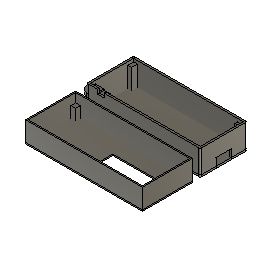
Asksin XS Board (Autodesk Fusion 360 design; units mm, degrees)
Autodesk Fusion 360 part; units mm, degrees
sketch "Skizze1" plane through (0, 0, 0) normal (0, 0, 1) x (1, 0, 0)
  line L0 (0.0871, 28.0002) -> (59.7871, 28.0002)
  line L1 (59.7871, 28.0002) -> (59.7871, 3.4002)
  line L2 (59.7871, 3.4002) -> (0.0871, 3.4002)
  line L3 (0.0871, 3.4002) -> (0.0871, 28.0002)
  line L4 (58.7871, 4.4002) -> (1.0871, 4.4002)
  line L5 (1.0871, 4.4002) -> (1.0871, 27.0002)
  line L6 (1.0871, 27.0002) -> (58.7871, 27.0002)
  line L7 (58.7871, 27.0002) -> (58.7871, 4.4002)
  line L8 (1.0871, 27.0002) -> (3.0871, 27.0002)
  line L9 (3.0871, 27.0002) -> (3.0871, 24.0002)
  line L10 (3.0871, 24.0002) -> (1.0871, 24.0002)
  line L11 (1.0871, 24.0002) -> (1.0871, 27.0002)
  line L12 (1.0871, 4.4002) -> (9.0871, 4.4002)
  line L13 (9.0871, 4.4002) -> (9.0871, 6.9002)
  line L14 (9.0871, 6.9002) -> (1.0871, 6.9002)
  line L15 (1.0871, 6.9002) -> (1.0871, 4.4002)
  line L16 (58.7871, 27.0002) -> (55.7871, 27.0002)
  line L17 (55.7871, 27.0002) -> (55.7871, 25.5002)
  line L18 (55.7871, 25.5002) -> (58.7871, 25.5002)
  line L19 (58.7871, 25.5002) -> (58.7871, 27.0002)
  line L20 (58.7871, 4.4002) -> (55.7871, 4.4002)
  line L21 (55.7871, 4.4002) -> (55.7871, 5.9002)
  line L22 (55.7871, 5.9002) -> (58.7871, 5.9002)
  line L23 (58.7871, 5.9002) -> (58.7871, 4.4002)
  line L24 (58.7871, 19.7002) -> (59.7871, 19.7002)
  line L25 (59.7871, 19.7002) -> (59.7871, 11.7002)
  line L26 (59.7871, 11.7002) -> (58.7871, 11.7002)
  line L27 (58.7871, 11.7002) -> (58.7871, 19.7002)
  circle A0 centre (-5.1629, 15.7002) radius 1.75
  line L28 (0.0871, 20.9502) -> (-6.9129, 20.9502)
  line L29 (-10.4129, 17.4502) -> (-10.4129, 13.9502)
  line L30 (-6.9129, 10.4502) -> (0.0871, 10.4502)
  line L31 (0.0871, 10.4502) -> (0.0871, 20.9502)
  arc A1 (-6.9129, 20.9502) -> (-10.4129, 17.4502) centre (-6.9129, 17.4502) ccw
  arc A2 (-10.4129, 13.9502) -> (-6.9129, 10.4502) centre (-6.9129, 13.9502) ccw
  point P0 (-10.4129, 20.9502)
  point P1 (-5.1629, 20.9502)
  point P2 (-10.4129, 15.7002)
  point P3 (0.0871, 15.7002)
  dimension "d1" = 59.7
  dimension "d2" = 24.6
  dimension "d3" = 1
  dimension "d4" = 2
  dimension "d5" = 3
  dimension "d6" = 8
  dimension "d7" = 2.5
  dimension "d8" = 3
  dimension "d9" = 1.5
  dimension "d10" = 3
  dimension "d11" = 1.5
  dimension "d12" = 1
  dimension "d13" = 8
  dimension "d14" = 8.3
  dimension "d57" = 3.5
  dimension "d58" = 10.5
  dimension "d59" = 10.5
  dimension "d60" = 3.5
  constraint horizontal L0
  constraint vertical L1
  constraint horizontal L2
  constraint vertical L3
  constraint horizontal L8
  constraint vertical L9
  constraint horizontal L10
  constraint vertical L11
  constraint horizontal L12
  constraint vertical L13
  constraint horizontal L14
  constraint vertical L15
  constraint horizontal L16
  constraint vertical L17
  constraint horizontal L18
  constraint vertical L19
  constraint horizontal L20
  constraint vertical L21
  constraint horizontal L22
  constraint vertical L23
  constraint horizontal L24
  constraint vertical L25
  constraint horizontal L26
  constraint vertical L27
  constraint coincident L7 L24.start
  constraint horizontal L28
  constraint vertical L29
  constraint horizontal L30
  constraint vertical L31
  constraint coincident L3 L28.start
  constraint vertical A0.centre P1
  constraint horizontal A0.centre P2
  constraint midpoint L3 P3
  constraint horizontal A0.centre P3
  constraint coincident L28 P1
  constraint coincident L29 P2
  constraint coincident P0 L28
  constraint coincident P0 L29
  constraint tangent L28 A1
  constraint tangent L29 A1
  constraint tangent L29 A2
  constraint tangent L30 A2
  constraint equal A1 A2
  measures "d1" distance of L0.start L0.end
  measures "d2" distance of L0.start L2.end
  measures "d4" distance of L5.end L8.end
  measures "d5" distance of L5.end L10.end
  measures "d6" distance of L4.end L12.end
  measures "d7" distance of L4.end L14.end
  measures "d8" distance of L6.end L16.end
  measures "d9" distance of L6.end L18.end
  measures "d10" distance of L4.start L20.end
  measures "d11" distance of L4.start L22.end
  measures "d12" distance of L24.start L24.end
  measures "d13" distance of L24.start L26.end
  measures "d14" distance of L0 L24
  measures "d57" diameter of A0
  measures "d58" distance of L28.start P0
  measures "d59" distance of L28.start L30.end
  measures "d60" radius of A1
extrude "Extrusion1" add sketch "Skizze1" along normal blind 1 contours L0 L1 L2 L3 L4 L5 L6 L7 L8 L11 L12 L15 L16 L19 L20 L23 L24 L26 L31 | L1 L7 L24 L25 L26 L27 | L4 L5 L6 L7 L9 L10 L13 L14 L17 L18 L21 L22 L27 | L6 L7 L16 L17 L18 L19 | L4 L7 L20 L21 L22 L23 | L5 L6 L8 L9 L10 L11 | L4 L5 L12 L13 L14 L15 makes body 1
extrude "Extrusion3" add sketch "Skizze1" along normal blind 13.2 separate body contours L0 L1 L2 L3 L4 L5 L6 L7 L8 L11 L12 L15 L16 L19 L20 L23 L24 L26 L31 | L1 L7 L24 L25 L26 L27 makes body 2
extrude "Extrusion4" cut sketch "Skizze1" along normal blind 5 contours L1 L7 L24 L25 L26 L27 bodies 2
sketch "Skizze2" plane through (0, 0, 0) normal (0, 0, 1) x (1, 0, 0)
  line L0 (59.9433, -27.2284) -> (-1.5067, -27.2284)
  line L1 (-1.5067, -27.2284) -> (-1.5067, -0.9284)
  line L2 (-1.5067, -0.9284) -> (59.9433, -0.9284)
  line L3 (59.9433, -0.9284) -> (59.9433, -27.2284)
  line L4 (-0.8067, -1.6284) -> (59.2433, -1.6284)
  line L5 (59.2433, -1.6284) -> (59.2433, -26.5284)
  line L6 (59.2433, -26.5284) -> (-0.8067, -26.5284)
  line L7 (-0.8067, -26.5284) -> (-0.8067, -1.6284)
  line L8 (26.7433, -9.5784) -> (51.7433, -9.5784)
  line L9 (51.7433, -9.5784) -> (51.7433, -18.5784)
  line L10 (51.7433, -18.5784) -> (26.7433, -18.5784)
  line L11 (26.7433, -18.5784) -> (26.7433, -9.5784)
  line L12 (-0.8067, -1.6284) -> (1.6933, -1.6284)
  line L13 (1.6933, -1.6284) -> (1.6933, -4.1284)
  line L14 (1.6933, -4.1284) -> (-0.8067, -4.1284)
  line L15 (-0.8067, -4.1284) -> (-0.8067, -1.6284)
  line L16 (-0.8067, -26.5284) -> (1.6933, -26.5284)
  line L17 (1.6933, -26.5284) -> (1.6933, -24.0284)
  line L18 (1.6933, -24.0284) -> (-0.8067, -24.0284)
  line L19 (-0.8067, -24.0284) -> (-0.8067, -26.5284)
  line L20 (59.2433, -1.6284) -> (56.7433, -1.6284)
  line L21 (56.7433, -1.6284) -> (56.7433, -4.1284)
  line L22 (56.7433, -4.1284) -> (59.2433, -4.1284)
  line L23 (59.2433, -4.1284) -> (59.2433, -1.6284)
  line L24 (59.2433, -26.5284) -> (56.7433, -26.5284)
  line L25 (56.7433, -26.5284) -> (56.7433, -24.0284)
  line L26 (56.7433, -24.0284) -> (59.2433, -24.0284)
  line L27 (59.2433, -24.0284) -> (59.2433, -26.5284)
  dimension "d23" = 61.45
  dimension "d24" = 26.3
  dimension "d26" = 0.7
  dimension "d27" = 25
  dimension "d28" = 9
  dimension "d29" = 8.65
  dimension "d30" = 7.5
  dimension "d37" = 2.5
  dimension "d38" = 2.5
  dimension "d39" = 2.5
  dimension "d40" = 2.5
  dimension "d41" = 2.5
  dimension "d42" = 2.5
  dimension "d43" = 2.5
  dimension "d44" = 2.5
  dimension "d63" = 24.5
  dimension "d64" = 59.5
  dimension "d65" = 7.4
  constraint horizontal L2
  constraint vertical L3
  constraint horizontal L0
  constraint vertical L1
  constraint horizontal L8
  constraint vertical L9
  constraint horizontal L10
  constraint vertical L11
  constraint horizontal L12
  constraint vertical L13
  constraint horizontal L14
  constraint vertical L15
  constraint horizontal L16
  constraint vertical L17
  constraint horizontal L18
  constraint vertical L19
  constraint horizontal L20
  constraint vertical L21
  constraint horizontal L22
  constraint vertical L23
  constraint horizontal L24
  constraint vertical L25
  constraint horizontal L26
  constraint vertical L27
  measures "d23" distance of L2.end L1.end
  measures "d24" distance of L1.end L0.end
  measures "d27" distance of L8.start L8.end
  measures "d28" distance of L8.start L10.end
  measures "d29" distance of L2 L8
  measures "d30" distance of L5 L9
  measures "d37" distance of L4.start L12.end
  measures "d38" distance of L4.start L14.end
  measures "d39" distance of L6.end L16.end
  measures "d40" distance of L6.end L18.end
  measures "d41" distance of L4.end L20.end
  measures "d42" distance of L4.end L22.end
  measures "d43" distance of L5.end L24.end
  measures "d44" distance of L5.end L26.end
extrude "Extrusion5" add sketch "Skizze2" along normal blind 0.7 separate body contours L0 L1 L2 L3 | L4 L7 L12 L13 L14 L15 | L4 L5 L6 L7 L13 L14 L17 L18 L21 L22 L25 L26 | L4 L5 L20 L21 L22 L23 | L6 L7 L16 L17 L18 L19 | L5 L6 L24 L25 L26 L27 makes body 3
extrude "Extrusion6" add sketch "Skizze2" along normal blind 11 separate body contours L0 L1 L2 L3 makes body 4
extrude "Extrusion7" add sketch "Skizze1" along normal blind 11.6 separate body contours L6 L7 L16 L17 L18 L19 | L4 L7 L20 L21 L22 L23 | L5 L6 L8 L9 L10 L11 | L4 L5 L12 L13 L14 L15 makes body 5 at (56.7871, 27.0002, 3.8667) makes body 6 at (57.7871, 4.4002, 3.8667) makes body 7 at (1.0871, 25.0002, 3.8667) makes body 8 at (6.4204, 6.9002, 3.8667)
extrude "Extrusion8" add sketch "Skizze2" along normal blind 6.3 separate body contours L4 L7 L12 L13 L14 L15 | L4 L5 L20 L21 L22 L23 | L6 L7 L16 L17 L18 L19 | L5 L6 L24 L25 L26 L27 makes body 9 at (0.0266, -1.6284, 2.1) makes body 10 at (0.86, -24.0284, 2.1) makes body 11 at (59.2433, -2.4617, 2.1) makes body 12 at (58.41, -26.5284, 2.1)
fillet "Abrundung1" radius 0.7 1 edges at (0.0871, 28.0002, 6.6) on bodies 2
fillet "Abrundung2" radius 0.7 1 edges at (0.0871, 28.0002, 0.5) on bodies 1
fillet "Abrundung3" radius 0.7 2 edges at (0.0871, 3.4002, 0.5) (0.0871, 3.4002, 6.6) on bodies 1 2
fillet "Abrundung4" radius 0.7 1 edges at (59.7871, 28.0002, 6.6) on bodies 2
fillet "Abrundung5" radius 0.7 1 edges at (59.7871, 28.0002, 0.5) on bodies 1
fillet "Abrundung6" radius 0.7 2 edges at (59.7871, 3.4002, 0.5) (59.7871, 3.4002, 6.6) on bodies 1 2
sketch "Skizze3" plane through (0, 3.4002, 0) normal (0, -1, 0) x (1, 0, 0)
  line L0 (59.0871, 0) -> (59.0871, 13.2)
  line L1 (59.0871, 13.2) -> (0.7871, 13.2)
  line L2 (0.7871, 13.2) -> (0.7871, 0)
  line L3 (0.7871, 0) -> (59.0871, 0)
  line L4 (9.1398, 13.2) -> (5.6398, 13.2)
  line L5 (5.6398, 13.2) -> (5.6398, 11)
  line L6 (5.6398, 11) -> (9.1398, 11)
  line L7 (9.1398, 11) -> (9.1398, 13.2)
  dimension "d53" = 3.5
  dimension "d54" = 2.2
  constraint horizontal L4
  constraint vertical L5
  constraint horizontal L6
  constraint vertical L7
  constraint coincident L1 L4.start
  measures "d53" distance of L4.start L4.end
  measures "d54" distance of L4.start L6.end
extrude "Extrusion9" cut sketch "Skizze3" against normal blind 4 contours L1 L4 L5 L6 L7 bodies 2 8
extrude "Extrusion10" add sketch "Skizze1" along normal blind 1.75 separate body contours L3 L28 L29 L30 L31 A1 A2 makes body 13
equation "d19 = 11.6 mm + 1.6 mm"
equation "d23 = 59.7 mm + 1.75 mm"
equation "d24 = 24.5 mm + 1.8 mm"
equation "d30 = 6.8 mm + 0.7 mm"
equation "d45 = 5.6 mm + 0.7 mm"
